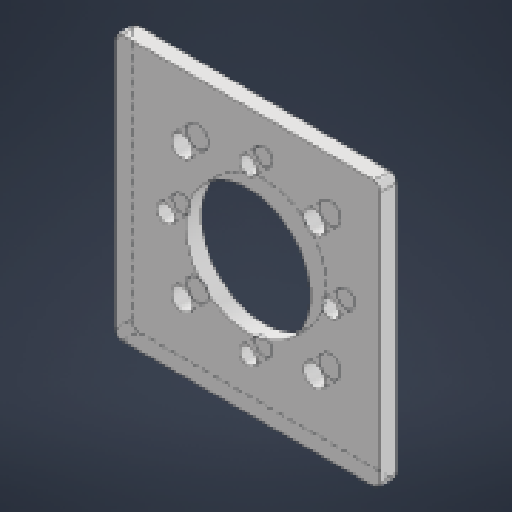
# Autodesk Inventor part: PL_BOTTOM
Saved by Autodesk Inventor 2023 (Build 270158000, 158)
## iProperties
Created: 2025-09-04
Part Number: PL_BOTTOM
Material: 일반
Document SubType Name: Modeling
Designer: k
Density: 1 g/cm^3
Appearance: 기본값
Author: k
Autodesk Inventor part; units mm, degrees
ref_plane "YZ Plane" through (0, 0, 0) normal (1, 0, 0) x (0, 1, 0)
ref_plane "XZ Plane" through (0, 0, 0) normal (0, 1, 0) x (-1, 0, 0)
ref_plane "XY Plane" through (0, 0, 0) normal (0, 0, 1) x (1, 0, 0)
sketch "스케치1" plane through (0, 0, 0) normal (0, 0, 1) x (1, 0, 0)
  line L0 (-70.5949, -22.2788) -> (24.4051, -22.2788)
  line L1 (26.9051, -24.7788) -> (26.9051, -119.7788)
  line L2 (24.4051, -122.2788) -> (-70.5949, -122.2788)
  line L3 (-73.0949, -119.7788) -> (-73.0949, -24.7788)
  circle A0 centre (-23.0949, -72.2788) radius 23.6
  circle A1 centre (-48.0949, -47.2788) radius 4.1
  circle A2 centre (1.9051, -47.2788) radius 4.1
  circle A3 centre (1.9051, -97.2788) radius 4.1
  circle A4 centre (-48.0949, -97.2788) radius 4.1
  circle A5 centre (-23.0949, -72.2788) radius 31
  circle A6 centre (-54.0949, -72.2788) radius 3.3
  circle A7 centre (-23.0949, -41.2788) radius 3.3
  circle A8 centre (7.9051, -72.2788) radius 3.3
  circle A9 centre (-23.0949, -103.2788) radius 3.3
  arc A10 (-70.5949, -22.2788) -> (-73.0949, -24.7788) centre (-70.5949, -24.7788) ccw
  arc A11 (-73.0949, -119.7788) -> (-70.5949, -122.2788) centre (-70.5949, -119.7788) ccw
  arc A12 (24.4051, -122.2788) -> (26.9051, -119.7788) centre (24.4051, -119.7788) ccw
  arc A13 (26.9051, -24.7788) -> (24.4051, -22.2788) centre (24.4051, -24.7788) ccw
  point P0 (0, 0)
  point P1 (26.9051, -122.2788)
  point P2 (26.9051, -22.2788)
  point P3 (-73.0949, -122.2788)
  dimension "d0" = 100
  dimension "d1" = 100
  dimension "d2" = 47.2
  dimension "d4" = 8.2
  dimension "d5" = 8.2
  dimension "d6" = 8.2
  dimension "d7" = 8.2
  dimension "d8" = 50
  dimension "d10" = 50
  dimension "d11" = 50
  dimension "d12" = 50
  dimension "d13" = 25
  dimension "d14" = 25
  dimension "d15" = 25
  dimension "d16" = 25
  dimension "d17" = 62
  dimension "d19" = 6.6
  dimension "d22" = 6.6
  dimension "d24" = 6.6
  dimension "d25" = 6.6
  dimension "d26" = 2.5
  constraints: 14 centre point, 12 point on circle, 8 end point, 8 tangent, 6 point on line, 3 equal radius, 2 parallel, 1 coincident, 1 horizontal, 1 perpendicular
  measures "d0" distance of point (26.905, -122.279) point (-73.095, -122.279)
  measures "d1" distance of point (26.905, -22.279) point (26.905, -122.279)
  measures "d2" diameter of A0
  measures "d4" diameter of A1
  measures "d5" diameter of A2
  measures "d6" diameter of A3
  measures "d7" diameter of A4
  measures "d8" distance of A4.centre A1.centre
  measures "d10" distance of A3.centre A4.centre
  measures "d11" distance of A2.centre A3.centre
  measures "d12" distance of A2.centre A1.centre
  measures "d13" distance from line of L0 A1.centre
  measures "d14" distance from line of L3 A1.centre
  measures "d15" distance from line of L1 A2.centre
  measures "d16" distance from line of L2 A4.centre
  measures "d17" diameter of A5
  measures "d19" diameter of A7
  measures "d22" diameter of A8
  measures "d24" diameter of A9
  measures "d25" diameter of A6
  measures "d26" radius of A10
extrude "돌출1" add sketch "스케치1" along normal blind 6 contours L0 A13 L1 A12 L2 A11 L3 A10 | A8 A5 A9 A6 A7
